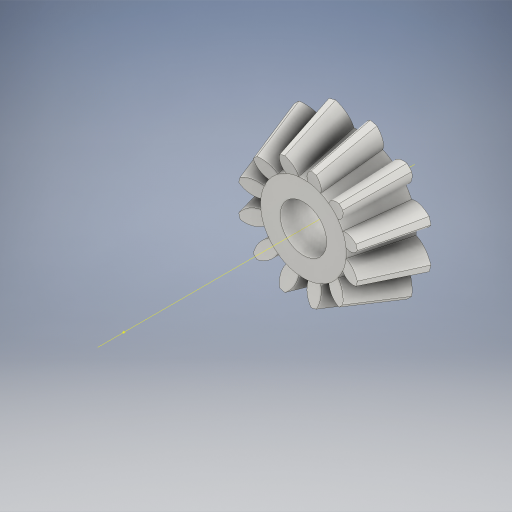
# Autodesk Inventor part: Bevel Gear1
Saved by Autodesk Inventor 2024 (Build 280153000, 153)
## iProperties
CustomPartVersion: 1
Created: 2024-04-12
Part Number: Bevel Gear1
Material: Steel, Mild
Document SubType Name: Modeling
Designer: Alex
Categories: <?xml version="1.0" encoding="UTF-16"?> <MemberInstance><Categories><FamilyTemplate><FamilyTemplateParameter ValueType="xs:double" Id="1" ObjectReferenceKey="da_z" ObjectType="kUserParameterObject"/><FamilyTemplateParameter ValueType="xs:double" Id="2" ObjectReferenceKey="da_b" ObjectType="kUserParameterObject"/><FamilyTemplateParameter ValueType="xs:double" Id="3" ObjectReferenceKey="da_beta" ObjectType="kUserParameterObject"/><FamilyTemplateParameter ValueType="xs:double" Id="4" ObjectReferenceKey="da_dae" ObjectType="kUserParameterObject"/><FamilyTemplateParameter ValueType="xs:double" Id="5" ObjectReferenceKey="da_ve" ObjectType="kUserParameterObject"/><FamilyTemplateParameter ValueType="xs:double" Id="6" ObjectReferenceKey="da_omega" ObjectType="kUserParameterObject"/><FamilyTemplateParameter ValueType="xs:string" Id="7" ObjectReferenceKey="EAIAABAAAAAAHwAAAAAAAIAAAAAAAAAA" ObjectType="83914240" SubObjectId="SurfaceGeometry"/></FamilyTemplate><ParamToTemplateMap><ParamToTemplate CategoryParameter="//CategoryParameter[@InternalName='046C89C9-8512-4d59-83FE-43B91F4F132A']" TemplateParameter="1"/><ParamToTemplate CategoryParameter="//CategoryParameter[@InternalName='2552DF32-E462-4b46-AEBF-C6C7768E72AC']" TemplateParameter="2"/><ParamToTemplate CategoryParameter="//CategoryParameter[@InternalName='C9EE641D-15FC-4fae-A226-E94C4372FDD7']" TemplateParameter="3"/><ParamToTemplate><ParamToTemplate CategoryParameter="//CategoryParameter[@InternalName='00B6519A-459B-49c7-AD84-2E56D39A5744']" ConstantValue="0.000000"/></ParamToTemplate><ParamToTemplate><ParamToTemplate CategoryParameter="//CategoryParameter[@InternalName='04B31F0E-C7A6-4894-AA32-9629BEFACF47']" ConstantValue="1.000000"/></ParamToTemplate><ParamToTemplate><ParamToTemplate CategoryParameter="//CategoryParameter[@InternalName='43CBEC2E-7847-49e7-A936-2F7889FCB2D9']" ConstantValue="0.200000"/></ParamToTemplate><ParamToTemplate><ParamToTemplate CategoryParameter="//CategoryParameter[@InternalName='B1EFC894-105D-4ebd-86BF-FA20ED196853']" ConstantValue="0.269800"/></ParamToTemplate><ParamToTemplate><ParamToTemplate CategoryParameter="//CategoryParameter[@InternalName='51175063-3D10-4879-93E8-6246FE8B403D']" ConstantValue="2060000000.000000"/></ParamToTemplate><ParamToTemplate><ParamToTemplate CategoryParameter="//CategoryParameter[@InternalName='A3A52E27-4454-46a9-B0BD-C932399B70AF']" ConstantValue="0.300000"/></ParamToTemplate><ParamToTemplate CategoryParameter="//CategoryParameter[@InternalName='2A200944-5A8C-41ca-B96E-8520D2E510F1']" TemplateParameter="4"/><ParamToTemplate><ParamToTemplate CategoryParameter="//CategoryParameter[@InternalName='1A637F62-92C8-44bc-B81F-10802510B579']" ConstantValue="2.090632"/></ParamToTemplate><ParamToTemplate CategoryParameter="//CategoryParameter[@InternalName='B52DD4BE-6863-48fb-BF58-89EF6F9EC65C']" TemplateParameter="5"/><ParamToTemplate><ParamToTemplate CategoryParameter="//CategoryParameter[@InternalName='3956BFF2-84D2-457d-93C2-9B0613DEBA67']" ConstantValue="3.002375"/></ParamToTemplate><ParamToTemplate CategoryParameter="//CategoryParameter[@InternalName='739CFA02-461B-4bf8-8049-181FCAD8B28F']" TemplateParameter="6"/><ParamToTemplate><ParamToTemplate CategoryParameter="//CategoryParameter[@InternalName='A27E999F-E2CE-4481-8A2A-EBF499C4C3C5']" ConstantValue="0.000000"/></ParamToTemplate><ParamToTemplate><ParamToTemplate CategoryParameter="//CategoryParameter[@InternalName='9E1B4470-B2D3-4ff1-B813-535BB4CDF51A']" ConstantValue="5000000.000000"/></ParamToTemplate><ParamToTemplate><ParamToTemplate CategoryParameter="//CategoryParameter[@InternalName='F8452263-BFF6-458c-9FB1-07C4B99E95CD']" ConstantValue="11400000.000000"/></ParamToTemplate><ParamToTemplate><ParamToTemplate CategoryParameter="//CategoryParameter[@InternalName='3E3BB259-FD49-497f-8171-6EBC954A3479']" ConstantValue="2.000000"/></ParamToTemplate><ParamToTemplate CategoryParameter="//CategoryParameter[@InternalName='27C3BAF2-7550-4e4b-AE2C-0DB134B7D9B7']" TemplateParameter="7"/></ParamToTemplateMap><Category DisplayName="Gear" InternalName="DC85795E-93AB-48d5-8EEE-5A27447B64BD" Mnemonic="Gear"><CategoryParameter DisplayName="z" InternalName="046C89C9-8512-4d59-83FE-43B91F4F132A" Mnemonic="z"/><CategoryParameter DisplayName="b" InternalName="2552DF32-E462-4b46-AEBF-C6C7768E72AC" Mnemonic="b"/><CategoryParameter DisplayName="||b|" InternalName="C9EE641D-15FC-4fae-A226-E94C4372FDD7" Mnemonic="beta"/><CategoryParameter DisplayName="x" InternalName="00B6519A-459B-49c7-AD84-2E56D39A5744" Mnemonic="x"/><CategoryParameter DisplayName="a*" InternalName="04B31F0E-C7A6-4894-AA32-9629BEFACF47" Mnemonic="a"/><CategoryParameter DisplayName="c*" InternalName="43CBEC2E-7847-49e7-A936-2F7889FCB2D9" Mnemonic="c"/><CategoryParameter DisplayName="r|.f|*" InternalName="B1EFC894-105D-4ebd-86BF-FA20ED196853" Mnemonic="rf"/><CategoryParameter DisplayName="E" InternalName="51175063-3D10-4879-93E8-6246FE8B403D" Mnemonic="E"/><CategoryParameter DisplayName="||m|" InternalName="A3A52E27-4454-46a9-B0BD-C932399B70AF" Mnemonic="mi"/><Category DisplayName="BevelGear" InternalName="0C98F69A-0C2B-4791-B2FE-7691BB227E77" Mnemonic="BevelGear"><CategoryParameter DisplayName="d|.ae|" InternalName="2A200944-5A8C-41ca-B96E-8520D2E510F1" Mnemonic="dae"/><CategoryParameter DisplayName="d|.ai|" InternalName="1A637F62-92C8-44bc-B81F-10802510B579" Mnemonic="dai"/><CategoryParameter DisplayName="A|.e|" InternalName="B52DD4BE-6863-48fb-BF58-89EF6F9EC65C" Mnemonic="ve"/><CategoryParameter DisplayName="A|.i|" InternalName="3956BFF2-84D2-457d-93C2-9B0613DEBA67" Mnemonic="vi"/><CategoryParameter DisplayName="||S|" InternalName="739CFA02-461B-4bf8-8049-181FCAD8B28F" Mnemonic="omega"/><CategoryParameter DisplayName="x|.t|" InternalName="A27E999F-E2CE-4481-8A2A-EBF499C4C3C5" Mnemonic="xt"/><CategoryParameter DisplayName="||s||.Flim|" InternalName="9E1B4470-B2D3-4ff1-B813-535BB4CDF51A" Mnemonic="sFlim"/><CategoryParameter DisplayName="||s||.Hlim|" InternalName="F8452263-BFF6-458c-9FB1-07C4B99E95CD" Mnemonic="sHlim"/><CategoryParameter DisplayName="type" InternalName="3E3BB259-FD49-497f-8171-6EBC954A3479" Mnemonic="type"/><CategoryParameter DisplayName="PitchDiameter" InternalName="27C3BAF2-7550-4e4b-AE2C-0DB134B7D9B7" Mnemonic="IDS_PITCHDIAM"/></Category></Category></Categories></MemberInstance>
Mass: 60.9118 g
Surface Area: 34.3074 cm^2
Volume: 7.7496 cm^3
Density: 7.86 g/cm^3
Appearance: Steel
Author: Alex
Autodesk Inventor part; units mm, degrees
ref_plane "Mesh Plane2" through (0, 0, 0) normal (0.9659258, 0.258819, 0) x (0, 0, 1)
sketch "Teeth Body Sketch" plane through (0, 0, 0) normal (1, 0, 0) x (0, 1, 0)
  line L0 (0, 0) -> (9.701217, -40.689635) construction
  line L1 (9.701217, -40.689635) -> (13.744331, -39.476701)
  line L2 (13.744331, -39.476701) -> (0, 0) construction
  line L3 (12, -40) -> (0, 0) construction
  line L4 (7.378197, -30.946234) -> (10.45316, -30.023745)
  line L5 (9.701217, -40.689635) -> (7.378197, -30.946234)
  line L6 (13.744331, -39.476701) -> (10.45316, -30.023745)
  line L7 (0, -39.386751) -> (0, 6.564458)
  line L8 (0, -40) -> (13.744331, -40) construction
  dimension "d0" = 24
  dimension "d1" = 19.40243
  dimension "d2" = 27.48866
  dimension "d3" = 10
  dimension "d4" = 39.4767
  constraints: 16 end point, 4 point on line, 3 perpendicular, 2 collinear, 1 horizontal alignment, 1 vertical alignment
  measures "d0" diameter of L3.start L7
  measures "d1" diameter of L0.end L7
  measures "d2" diameter of L1.end L7
  measures "d3" distance between parallel lines of L1 L4
  measures "d4" vertical distance of L1.end L0.start
revolve "Teeth Body" add sketch "Teeth Body Sketch" angle 360 about axis through (0, 0, 0) along (0, 0, 1)
ref_plane "Tooth Plane" through (0, 12, -40) normal (0, -0.2873479, 0.9578263) x (1, 0, 0)
sketch "Start Sketch" plane through (0, 12, -40) normal (0, -0.2873479, 0.9578263) x (1, 0, 0)
  line L0 (0, -23.505131) -> (0, 10.644758)
  arc A0 (-1.08702, -2.906536) -> (-4.874233, 2.307278) centre (-5.702944, -2.277067) ccw
  arc A1 (4.874233, 2.307278) -> (1.08702, -2.906536) centre (5.702944, -2.277067) ccw
  line L1 (-1.08702, -2.906536) -> (1.08702, -2.906536)
  arc A2 (4.874233, 2.307278) -> (-4.874233, 2.307278) centre (0, -12.528368) ccw
  dimension "d7" = 4.65865
  dimension "d8" = 5.70294
  dimension "d9" = 10.2513
  dimension "d57" = 15.61584
  dimension "d58" = 9.62183
  constraints: 6 point on circle, 3 centre point, 3 symmetric about line, 2 end point, 1 coincident, 1 perpendicular, 1 other
  measures "d7" radius of A0
  measures "d8" horizontal distance of point (0, -12.528) A0.centre
  measures "d9" vertical distance of point (0, -12.528) A0.centre
  measures "d57" radius of A2
  measures "d58" distance from line of A2.centre L1
sketch "End Sketch" plane through (0, 9.065874, -30.219581) normal (0, -0.2873479, 0.9578263) x (1, 0, 0)
  line L0 (0, -15.35404) -> (0, 6.953444)
  arc A0 (-0.821232, -2.195858) -> (-3.682432, 1.743125) centre (-4.308514, -1.7203) ccw
  arc A1 (3.682432, 1.743125) -> (0.821232, -2.195858) centre (4.308514, -1.7203) ccw
  line L1 (-0.821232, -2.195858) -> (0.821232, -2.195858)
  arc A2 (3.682432, 1.743125) -> (-3.682432, 1.743125) centre (0, -9.465051) ccw
  dimension "d12" = 3.51956
  dimension "d15" = 4.30851
  dimension "d16" = 7.74475
  dimension "d59" = 11.79761
  dimension "d60" = 7.26919
  constraints: 6 point on circle, 3 centre point, 3 symmetric about line, 2 end point, 1 coincident, 1 other
  measures "d12" radius of A0
  measures "d15" horizontal distance of A0.centre point (0, -9.465)
  measures "d16" vertical distance of A0.centre point (0, -9.465)
  measures "d59" radius of A2
  measures "d60" distance from line of A2.centre L1
loft "Loft" cut profiles "Start Sketch", "End Sketch"
pattern_circular "Circular Pattern" count 12 over 360 about axis through (0, 0, 0) along (0, 0, 1) of "Loft"
ref_plane "End Plane" through (0, 9.065874, -30.219581) normal (0, -0.2873479, 0.9578263) x (1, 0, 0)
sketch3d "3D Sketch Right"
ref_plane "End Plane Right" through (-3.124287, 8.510518, -30.219581) normal (0.099026, -0.2697455, 0.9578263) x (0.938742, 0.3446206, 0)
sketch "End Sketch Right" plane through (-3.124287, 8.510518, -30.219581) normal (0.099026, -0.2697455, 0.9578263) x (0.938742, 0.3446206, 0)
  arc A0 (-0.821232, -2.195858) -> (-3.682432, 1.743125) centre (-4.308514, -1.7203) ccw
  line L0 (0, -21.070417) -> (0, 12.66981)
  arc A1 (3.682432, 1.743125) -> (0.821232, -2.195858) centre (4.308514, -1.7203) ccw
  line L1 (-0.821232, -2.195858) -> (0.821232, -2.195858)
  arc A2 (3.682432, 1.743125) -> (-3.682432, 1.743125) centre (0, -9.465051) ccw
  dimension "d70" = 4.30851
  dimension "d71" = 7.74475
  dimension "d72" = 3.51956
  dimension "d73" = 7.26919
  dimension "d74" = 11.79761
  constraints: 6 point on circle, 3 centre point, 3 symmetric about line, 2 end point, 1 coincident, 1 perpendicular, 1 other
  measures "d70" horizontal distance of A2.centre A0.centre
  measures "d71" vertical distance of point (0, -9.465) A0.centre
  measures "d72" radius of A0
  measures "d73" distance from line of point (0, -9.465) L1
  measures "d74" radius of A2
feature "Loft Right" [suppressed]
pattern_circular "Circular Pattern Right" [suppressed]
sketch3d "3D Sketch Left"
ref_plane "End Plane Left" through (3.117559, 8.510518, -30.217435) normal (-0.0988213, -0.2697688, 0.9578409) x (0.938982, -0.3439663, 0)
sketch "End Sketch Left" plane through (3.117559, 8.510518, -30.217435) normal (-0.0988213, -0.2697688, 0.9578409) x (0.938982, -0.3439663, 0)
  line L0 (0, -37.093728) -> (0, 20.071005)
  arc A0 (-0.821232, -2.194255) -> (-3.682432, 1.744727) centre (-4.308514, -1.718698) ccw
  arc A1 (3.682432, 1.744727) -> (0.821232, -2.194255) centre (4.308514, -1.718698) ccw
  line L1 (-0.821232, -2.194255) -> (0.821232, -2.194255)
  ellipse E0 centre (0, -8.625799) end of major axis (10.45316, -8.625799) minor radius 10.012464
  arc A2 (3.682432, 1.744727) -> (-3.682432, 1.744727) centre (0, -9.463449) ccw
  dimension "d56" = 10.01246
  dimension "d30" = 3.51956
  dimension "d31" = 4.30851
  dimension "d32" = 7.74475
  dimension "d61" = 11.79761
  dimension "d62" = 7.26919
  constraints: 6 point on circle, 3 centre point, 3 symmetric about line, 2 end point, 1 coincident, 2 other
  measures "d30" radius of A0
  measures "d31" horizontal distance of point (0, -9.463) A0.centre
  measures "d32" vertical distance of A0.centre point (0, -9.463)
  measures "d61" radius of A2
  measures "d62" distance from line of point (0, -9.463) L1
feature "Loft Left" [suppressed]
pattern_circular "Circular Pattern Left" [suppressed]
sketch "Body Sketch" plane through (0, 0, 0) normal (1, 0, 0) x (0, 1, 0)
  line L0 (0, -35.037536) -> (0, -19.530831)
  line L1 (9.701217, -40.689635) -> (7.378197, -30.946234)
  line L2 (7.378197, -30.946234) -> (0, -30.946234)
  line L3 (9.701217, -40.689635) -> (0, -40.689635)
  constraints: 4 end point, 2 perpendicular, 2 point on line
sketch "Body Sketch outline for Fix Body" plane through (0, 0, 0) normal (1, 0, 0) x (0, 1, 0)
  line L0 (0, -40.689635) -> (9.701217, -40.689635)
  line L1 (0, -30.946234) -> (0, -40.689635)
  line L2 (7.378197, -30.946234) -> (0, -30.946234)
  line L3 (9.701217, -40.689635) -> (7.378197, -30.946234)
revolve "Fix Body" add sketch "Body Sketch outline for Fix Body" angle 360 about axis through (0, 0, 0) along (0, 0, 1)
sketch "Sketch6" plane through (0, 0, 0) normal (1, 0, 0) x (0, 1, 0)
  line L0 (12, -40) -> (0, 0)
  line L1 (0, -37.799919) -> (0, 6.299986)
surface revolve "Pitch Diameter" sketch "Sketch6" angle 360 about axis through (0, 0, 0) along (0, 0, 1) shown no curves L0
sketch "Sketch8" plane through (0, 0, -30.946234) normal (0, 0, 1) x (1, 0, 0)
  circle A0 centre (0, 0) radius 4
  dimension "d98" = 8
  constraints: 1 centre point
  measures "d98" diameter of A0
extrude "Extrusion1" cut sketch "Sketch8" against normal up to next
equation "\"d0\" = da_de"
equation "\"d1\" = da_dfe"
equation "\"d2\" = da_dae"
equation "\"d3\" = da_b"
equation "\"d4\" = da_ve"
equation "\"d7\" = fd_rr"
equation "\"d8\" = fd_x"
equation "\"d9\" = fd_y"
equation "\"d57\" = 0.5 * fd_dva + 0.3 * da_he"
equation "\"d58\" = 0.5 * fd_dva - 1.12 * da_he"
equation "\"da_teethtype\" = 0"
equation "\"da_b\" = 10"
equation "\"da_de\" = 24"
equation "\"da_dae\" = 27.48866"
equation "\"da_dfe\" = 19.40243"
equation "\"da_le\" = 41.76123"
equation "\"da_omega\" = 90deg"
equation "\"da_beta\" = 0"
equation "\"da_delta\" = 16.699244deg"
equation "\"da_alpha\" = 20deg"
equation "\"da_he\" = 4.22113"
equation "\"da_ve\" = 39.4767"
equation "\"da_zv\" = 12.528368"
equation "\"fd_loft\" = da_b + 0.05 * da_he"
equation "\"fd_x\" = fd_x1 + fd_x2"
equation "\"fd_y\" = fd_y1 - fd_y2"
equation "\"fd_dd\" = fd_dva - 0.8 * da_he"
equation "\"da_dvw\" = 25.05674"
equation "\"d11\" = fd_loft"
equation "\"da_dm\" = 21.12652"
equation "\"da_x\" = 0"
equation "\"da_m\" = 2"
equation "\"d50\" = da_omega"
equation "\"fd_rr\" = 4.658646"
equation "\"fd_dva\" = 28.699005"
equation "\"fd_x1\" = 1.583999"
equation "\"fd_x2\" = 4.118945"
equation "\"fd_y1\" = 12.42783"
equation "\"fd_y2\" = 2.176529"
body "Solid1"
body "Srf1"
